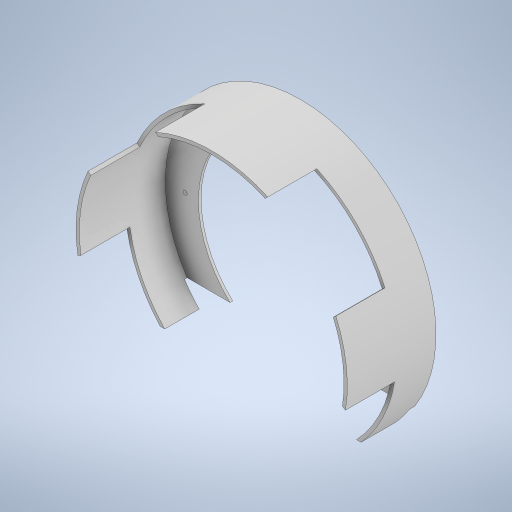
# Autodesk Inventor part: Falda-Parte1
Saved by Autodesk Inventor 2024.2 (Build 282272000, 272)
## iProperties
Created: 2023-12-12
Part Number: Falda-Parte1
Material: Generic
Document SubType Name: Modeling
Designer: felip
Density: 1 g/cm^3
Appearance: Default
Author: felip
Autodesk Inventor part; units mm, degrees
ref_plane "YZ Plane" through (0, 0, 0) normal (1, 0, 0) x (0, 1, 0)
ref_plane "XZ Plane" through (0, 0, 0) normal (0, 1, 0) x (-1, 0, 0)
ref_plane "XY Plane" through (0, 0, 0) normal (0, 0, 1) x (1, 0, 0)
sketch "Sketch1" plane through (0, 0, 0) normal (0, 0, 1) x (1, 0, 0)
  arc A0 (72.4335, -68.9449) -> (-72.4335, -68.9449) centre (0, 0) ccw
  line L0 (0, 0) -> (0, -68.9449)
  arc A1 (75.8476, -68.9449) -> (-75.8476, -68.9449) centre (0, 0) ccw
  line L1 (0, 0) -> (88.7676, -51.25)
  line L2 (0, 0) -> (102.5, 0) construction
  line L3 (0, 0) -> (-88.7676, -51.25)
  line L4 (0, 0) -> (102.5, 0) construction
  line L5 (0, 0) -> (72.4784, 72.4784)
  line L6 (0, 0) -> (102.5, 0) construction
  line L7 (0, 0) -> (-72.4784, 72.4784)
  line L8 (0, 0) -> (102.5, 0) construction
  line L9 (0, 0) -> (-68.416, -39.5)
  line L10 (0, 0) -> (68.416, -39.5)
  line L11 (0, 0) -> (55.8614, 55.8614)
  line L12 (0, 0) -> (-55.8614, 55.8614)
  line L13 (-68.416, -39.5) -> (-51.416, -68.9449)
  line L14 (-68.416, -39.5) -> (-85.416, -10.0551)
  line L15 (68.416, -39.5) -> (51.416, -68.9449)
  line L16 (51.416, -68.9449) -> (68.416, -39.5)
  line L17 (68.416, -39.5) -> (85.416, -10.0551)
  line L18 (-51.416, -68.9449) -> (-75.8476, -68.9449)
  line L19 (-51.416, -68.9449) -> (51.416, -68.9449)
  line L20 (51.416, -68.9449) -> (75.8476, -68.9449)
  line L21 (85.416, -10.0551) -> (100.7418, -18.9035)
  line L22 (-85.416, -10.0551) -> (-100.7418, -18.9035)
  line L23 (-55.8614, 55.8614) -> (-79.9031, 31.8198)
  line L24 (-55.8614, 55.8614) -> (-31.8198, 79.9031)
  line L25 (55.8614, 55.8614) -> (79.9031, 31.8198)
  line L26 (55.8614, 55.8614) -> (31.8198, 79.9031)
  line L27 (-31.8198, 79.9031) -> (-44.3333, 92.4165)
  line L28 (-79.9031, 31.8198) -> (-92.4165, 44.3333)
  line L29 (31.8198, 79.9031) -> (44.3333, 92.4165)
  line L30 (79.9031, 31.8198) -> (92.4165, 44.3333)
  circle A2 centre (0, 0) radius 125
  line L31 (100.7418, -18.9035) -> (121.1717, -30.6987)
  line L32 (-100.7418, -18.9035) -> (-121.1717, -30.6987)
  line L33 (-92.4165, 44.3333) -> (-109.0975, 61.0142)
  line L34 (-44.3333, 92.4165) -> (-61.0142, 109.0975)
  line L35 (44.3333, 92.4165) -> (61.0142, 109.0975)
  line L36 (92.4165, 44.3333) -> (109.0975, 61.0142)
  circle A3 centre (0, 0) radius 120
  line L37 (-75.8476, -68.9449) -> (-104.267, -68.9449)
  line L38 (75.8476, -68.9449) -> (104.267, -68.9449)
  line L39 (68.416, -39.5) -> (86.416, -8.3231)
  line L40 (86.416, -8.3231) -> (121.6665, -28.675)
  line L41 (55.8614, 55.8614) -> (81.3173, 30.4056)
  line L42 (81.3173, 30.4056) -> (111.6152, 56.2764)
  line L43 (-68.416, -39.5) -> (-86.416, -8.3231)
  line L44 (-86.416, -8.3231) -> (-121.6665, -28.675)
  line L45 (-55.8614, 55.8614) -> (-81.3173, 30.4056)
  line L46 (-81.3173, 30.4056) -> (-110.0992, 59.1875)
  line L47 (-55.8614, 55.8614) -> (-30.4056, 81.3173)
  line L48 (-30.4056, 81.3173) -> (-59.1875, 110.0992)
  line L49 (55.8614, 55.8614) -> (30.4056, 81.3173)
  line L50 (30.4056, 81.3173) -> (59.1875, 110.0992)
  line L51 (68.416, -39.5) -> (50.416, -70.6769)
  line L52 (-68.416, -39.5) -> (-50.416, -70.6769)
  line L53 (51.416, -68.9449) -> (87.1717, -89.5884)
  line L54 (51.416, -68.9449) -> (92.7032, -68.9449) construction
  line L55 (50.416, -70.6769) -> (85.6665, -91.0288)
  line L56 (-50.416, -70.6769) -> (-85.6665, -91.0288)
  line L57 (-51.416, -68.9449) -> (-87.1717, -89.5884)
  point P0 (93.8835, 41.1356)
  point P1 (91.8949, 39.4376)
  point P2 (98.796, -15.4707)
  point P3 (101.1125, -16.8081)
  point P4 (40.5138, 91.4255)
  point P5 (42.4052, 93.3169)
  point P6 (-42.4052, 93.3169)
  point P7 (-40.5138, 91.4255)
  point P8 (-91.4255, 40.5138)
  point P9 (-93.3169, 42.4052)
  point P10 (-101.1125, -16.8081)
  point P11 (-98.796, -15.4707)
  point P12 (98.2171, -68.9449)
  point P13 (98.4432, -17.5764)
  point P14 (116.6644, -28.0964)
  point P15 (57.334, 105.4173)
  point P16 (105.4173, 57.334)
  point P17 (-105.4173, 57.334)
  point P18 (-57.334, 105.4173)
  point P19 (-98.2171, -68.9449)
  point P20 (-116.6644, -28.0964)
  point P21 (90.5398, 42.4565)
  point P22 (42.4565, 90.5398)
  point P23 (-42.4565, 90.5398)
  point P24 (-90.5398, 42.4565)
  point P25 (-98.4432, -17.5764)
  point P26 (-86.6025, -50)
  point P27 (-82.6644, -86.9862)
  point P28 (82.6644, -86.9862)
  dimension "d30" = 250
  dimension "d7" = 30
  dimension "d8" = 150
  dimension "d9" = 45
  dimension "d10" = 135
  dimension "d11" = 79
  dimension "d12" = 79
  dimension "d13" = 79
  dimension "d14" = 79
  dimension "d15" = 34
  dimension "d16" = 90
  dimension "d17" = 34
  dimension "d18" = 34
  dimension "d19" = 34
  dimension "d20" = 34
  dimension "d21" = 34
  dimension "d22" = 34
  dimension "d23" = 34
  dimension "d24" = 34
  dimension "d31" = 240
  dimension "d32" = 36
  dimension "d33" = 36
  dimension "d34" = 36
  dimension "d35" = 36
  dimension "d36" = 36
  dimension "d37" = 36
  dimension "d73" = 36
  dimension "d74" = 36
  dimension "d75" = 30
  constraints: 116 end point, 16 point on line, 11 perpendicular, 10 equal length, 7 horizontal, 4 coincident, 2 centre point, 2 point on circle, 1 midpoint, 1 vertical, 34 other
  measures "d7" angle of L1 L2
  measures "d8" angle of L3 L4
  measures "d9" angle of L6 L5
  measures "d10" angle of L8 L7
  measures "d11" distance of L1.start L9.end
  measures "d12" distance of L1.start L10.end
  measures "d13" distance of L1.start L11.end
  measures "d14" distance of L1.start L12.end
  measures "d15" distance of L9.end L13.end
  measures "d16" angle of L9 L13
  measures "d17" distance of L9.end L14.end
  measures "d18" distance of L10.end L15.end
  measures "d19" distance of L15.end L10.end
  measures "d20" distance of L10.end L17.end
  measures "d21" distance of L12.end L23.end
  measures "d22" distance of L12.end L24.end
  measures "d23" distance of L11.end L25.end
  measures "d24" distance of L11.end L26.end
  measures "d31" diameter of A3
  measures "d32" distance of L10.end L39.end
  measures "d33" distance of L11.end L41.end
  measures "d34" distance of L9.end L43.end
  measures "d35" distance of L12.end L45.end
  measures "d36" distance of L12.end L47.end
  measures "d37" distance of L11.end L49.end
  measures "d73" distance of L10.end L51.end
  measures "d74" distance of L9.end L52.end
  measures "d75" angle of L53 L54
extrude "Extrusion3" add sketch "Sketch1" against normal blind 2 contours L20 L15 L1 A0 | A0 L1 A1 L20 | L1 L17 L21 A0 | A0 L21 A1 L1 | L19 L0 L1 L15 | L21 L39 L40 A0 | A0 L40 A1 L21 | L1 L5 L25 L41 L42 A0 L40 L39 L17 | L19 L13 L3 L0 | A0 L42 A1 L40 | L7 L24 L47 L48 A0 L50 L49 L26 L5 | L3 L14 L43 L44 A0 L46 L45 L23 L7 | L18 A0 L3 L13 | L42 L41 L30 A0 | A0 L30 A1 L42 | L3 A0 L22 L14 | L26 L29 A0 L5 | L5 A0 L30 L25 | L23 L28 A0 L7 | L7 A0 L27 L24 | L18 A1 L3 A0 | A0 L5 A1 L30 | L3 A1 L22 A0 | L22 A0 L44 L43 | A0 L29 A1 L5 | L49 L50 A0 L29 | L7 A1 L27 A0 | A0 L28 A1 L7 | L45 L46 A0 L28 | L27 A0 L48 L47 | L22 A1 L44 A0 | A0 L50 A1 L29 | L27 A1 L48 A0 | A0 L46 A1 L28 | L44 A1 L46 A0 | A0 L48 A1 L50
extrude "Extrusion4" add sketch "Sketch1" along normal blind 28 contours A0 L1 A1 L20 | A0 L21 A1 L1 | A0 L40 A1 L21 | A0 L42 A1 L40 | A0 L30 A1 L42 | L18 A1 L3 A0 | A0 L5 A1 L30 | L3 A1 L22 A0 | A0 L29 A1 L5 | L7 A1 L27 A0 | A0 L28 A1 L7 | L22 A1 L44 A0 | A0 L50 A1 L29 | L27 A1 L48 A0 | A0 L46 A1 L28 | L44 A1 L46 A0 | A0 L48 A1 L50
extrude "Extrusion5" add sketch "Sketch1" along normal blind 65 contours A0 L42 A1 L40 | L44 A1 L46 A0 | A0 L48 A1 L50
sketch "Sketch4" plane through (0, 0, -2) normal (0, 0, -1) x (-1, 0, 0)
  line L0 (0, 0) -> (-85, 0)
  line L1 (0, 0) -> (0, 85)
  line L2 (0, 0) -> (85, 0)
  circle A0 centre (-85, 0) radius 1.5
  circle A1 centre (0, 85) radius 1.5
  circle A2 centre (85, 0) radius 1.5
  circle A3 centre (0, 0) radius 75
  dimension "d60" = 85
  dimension "d61" = 85
  dimension "d62" = 85
  dimension "d63" = 3
  dimension "d64" = 3
  dimension "d65" = 3
  dimension "d66" = 150
  constraints: 6 end point, 4 centre point, 4 coincident, 2 horizontal, 1 vertical
  measures "d60" distance of L0.start L0.end
  measures "d61" distance of L0.start L1.end
  measures "d62" distance of L0.start L2.end
  measures "d63" diameter of A0
  measures "d64" diameter of A1
  measures "d65" diameter of A2
  measures "d66" diameter of A3
extrude "Extrusion11" cut sketch "Sketch4" against normal blind 45
sketch "Sketch5" plane through (0, 0, -2) normal (0, 0, -1) x (-1, 0, 0)
  line L0 (72.4335, -68.9449) -> (-72.4335, -68.9449) projected
  line L1 (-72.4335, -68.9449) -> (-72.4335, -54.9449)
  line L2 (-72.4335, -54.9449) -> (129.3344, -54.9449)
  line L3 (129.3344, -54.9449) -> (-118.857, -54.9449)
  line L4 (-118.857, -54.9449) -> (-118.857, -84.9238)
  line L5 (-118.857, -84.9238) -> (129.3344, -84.9238)
  line L6 (129.3344, -84.9238) -> (129.3344, -54.9449)
  point P0 (0, 0)
  point P1 (-41.6566, -68.9449)
  dimension "d70" = 14
  constraints: 12 end point, 2 parallel, 2 perpendicular, 1 horizontal, 1 vertical
  measures "d70" distance of L0.end L1.end
extrude "Extrusion12" cut sketch "Sketch5" against normal blind 4
body "Solid2"
